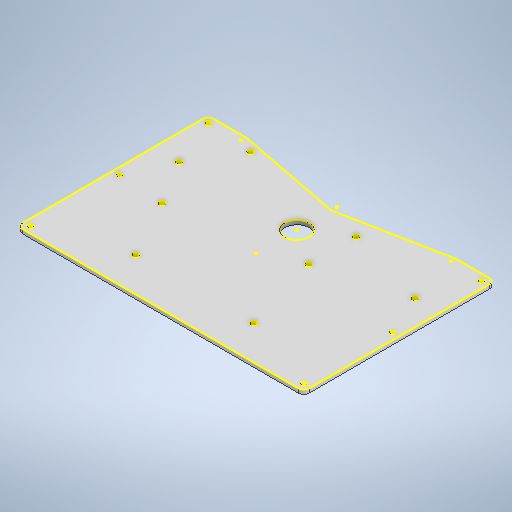
# Autodesk Inventor part: ローラー_板
Saved by Autodesk Inventor 2025.1 (Build 291241000, 241)
## iProperties
Created: 2024-10-14
Part Number: ローラー_板
Material: 一般
Document SubType Name: Modeling
Designer: taiju
Density: 1 g/cm^3
Appearance: 既定
Author: taiju
Autodesk Inventor part; units mm, degrees
ref_plane "YZ Plane" through (0, 0, 0) normal (1, 0, 0) x (0, 1, 0)
ref_plane "XZ Plane" through (0, 0, 0) normal (0, 1, 0) x (-1, 0, 0)
ref_plane "XY Plane" through (0, 0, 0) normal (0, 0, 1) x (1, 0, 0)
sketch "スケッチ1" plane through (0, 0, 0) normal (0, 1, 0) x (-1, 0, 0)
  line L0 (105, 70) -> (-105, 70)
  line L1 (-105, 70) -> (-105, -70)
  line L2 (-105, -70) -> (105, -70)
  line L3 (105, -70) -> (105, 70)
  line L4 (105, 70) -> (-105, -70) construction
  line L5 (-105, 70) -> (105, -70) construction
  circle A0 centre (0, -30) radius 77
  circle A1 centre (0, -30) radius 9
  line L6 (-105, -30) -> (105, -30)
  circle A2 centre (48, -30) radius 12.5
  circle A3 centre (-39, -30) radius 6
  circle A4 centre (48, -30) radius 17.5
  circle A5 centre (-39, -30) radius 9
  circle A6 centre (0, -30) radius 86.5
  line L7 (66.5, -30) -> (66.5, -62.5)
  line L8 (66.5, -30) -> (66.5, 2.5)
  line L9 (-26, -30) -> (-26, -47.5)
  line L10 (-26, -30) -> (-26, -12.5)
  circle A7 centre (65.5, -30) radius 2
  circle A8 centre (48, -12.5) radius 2
  circle A9 centre (30.5, -30) radius 2
  circle A10 centre (48, -47.5) radius 2
  circle A11 centre (-39, -39) radius 1.6
  circle A12 centre (-39, -21) radius 1.6
  circle A13 centre (-26, -47.5) radius 2
  circle A14 centre (-26, -12.5) radius 2
  circle A15 centre (66.5, -62.5) radius 2
  circle A16 centre (66.5, 2.5) radius 2
  circle A17 centre (86.5, -30) radius 2
  circle A18 centre (43.25, 44.9112) radius 2
  circle A19 centre (-43.25, 44.9112) radius 2
  circle A20 centre (-86.5, -30) radius 2
  line L11 (76.6958, -70) -> (0, -55)
  line L12 (0, -55) -> (-76.6958, -70)
  line L13 (100, -70) -> (100, 70)
  line L14 (-100, -70) -> (-100, 70)
  point P0 (0, 0)
  point P1 (-43.25, -104.9112)
  point P2 (43.25, -104.9112)
  point P3 (100, -65)
  point P4 (100, 0)
  point P5 (100, 65)
  point P6 (-100, -65)
  point P7 (-100, 0)
  point P8 (-100, 65)
  dimension "d9" = 35
  dimension "d0" = 210
  dimension "d1" = 140
  dimension "d2" = 100
  dimension "d3" = 154
  dimension "d4" = 18
  dimension "d5" = 48
  dimension "d6" = 39
  dimension "d7" = 25
  dimension "d8" = 12
  dimension "d10" = 18
  dimension "d11" = 173
  dimension "d14" = 360
  dimension "d16" = 18.5
  dimension "d17" = 32.5
  dimension "d18" = 32.5
  dimension "d20" = 13
  dimension "d21" = 17.5
  dimension "d22" = 17.5
  dimension "d25" = 360
  dimension "d27" = 4
  dimension "d28" = 4
  dimension "d29" = 4
  dimension "d30" = 4
  dimension "d31" = 3.2
  dimension "d32" = 3.2
  dimension "d33" = 4
  dimension "d34" = 4
  dimension "d35" = 4
  dimension "d36" = 4
  dimension "d37" = 4
  dimension "d38" = 4
  dimension "d39" = 4
  dimension "d40" = 4
  dimension "d41" = 15
  dimension "d45" = 5
  dimension "d46" = 5
  dimension "d47" = 5
  dimension "d48" = 5
  dimension "d49" = 5
  dimension "d50" = 5
  dimension "d51" = 5
  dimension "d52" = 5
  constraints: 30 end point, 26 coincident, 20 centre point, 17 point on line, 5 midpoint, 5 point on circle, 4 vertical, 2 parallel, 2 perpendicular, 1 horizontal, 1 horizontal alignment, 14 other
  measures "d0" distance of L2.end L1.end
  measures "d1" distance of L0.end L1.end
  measures "d2" distance from line of point (0, -30) L0
  measures "d3" diameter of A0
  measures "d4" diameter of A1
  measures "d5" distance of point (48, -30) point (0, -30)
  measures "d6" distance of point (-39, -30) point (0, -30)
  measures "d7" diameter of A2
  measures "d8" diameter of A3
  measures "d10" diameter of A5
  measures "d11" diameter of A6
  measures "d16" distance of L7.start point (48, -30)
  measures "d17" distance of L7.start L7.end
  measures "d18" distance of L7.start L8.end
  measures "d20" distance of L9.start A5.centre
  measures "d21" distance of L9.start L9.end
  measures "d22" distance of L9.start L10.end
  measures "d27" diameter of A7
  measures "d28" diameter of A8
  measures "d29" diameter of A9
  measures "d30" diameter of A10
  measures "d31" diameter of A11
  measures "d32" diameter of A12
  measures "d33" diameter of A13
  measures "d34" diameter of A14
  measures "d35" diameter of A15
  measures "d36" diameter of A16
  measures "d37" diameter of A17
  measures "d38" diameter of A18
  measures "d39" diameter of A19
  measures "d40" diameter of A20
  measures "d41" distance from line of L11.end L2
  measures "d45" distance from line of L13.start L3
  measures "d46" distance from line of L13.end L3
  measures "d47" distance from line of L14.start L1
  measures "d48" distance from line of L14.end L1
  measures "d49" distance from line of point (100, -65) L2
  measures "d50" distance from line of point (100, 65) L0
  measures "d51" distance from line of point (-100, -65) L2
  measures "d52" distance from line of point (-100, 65) L0
extrude "押し出し1" add sketch "スケッチ1" along normal blind 3 contours L3 L6 L13 L0 | L13 L6 A17 A6 A18 A19 A20 L14 L0 | L3 L2 L13 L6 | L14 L6 L1 L0 | L13 L2 A6 A17 L6 | L14 L2 L1 L6 | L6 A20 A6 L2 L14 | A17 L6 A0 A20 A6 A19 A18 | A6 L11 A0 L6 A17 | A20 L6 A0 L12 A6 | L11 L12 A0 L6 A5 A11 A1 A9 A4 A10 A7 | L6 A7 A4 A8 A9 A1 A5 A12 A0 | A7 L7 L6 | L6 L8 A7 | A5 A12 L6 A3 | L6 A3 A5 A11 | L7 A7 A4 L6 | L6 A4 A7 L8 | A3 L6 | L6 A3 | A12 A5 | A5 A12 | A11 A5 | A5 A11 | A4 A7 L6 | L6 A7 A4 | A7 L6 A2 A9 A4 A8 | A4 A10 A9 L6 A2 A7 | A8 A4 | A4 A8 | A10 A4 | A4 A10 | A2 L6 | L6 A2 | A9 L6 A4 | A4 L6 A9 | A9 L6 A4 | A4 L6 A9
fillet "フィレット1" radius 4 7 edges at (-105, 1.5, 70) (-105, 1.5, -70) (-76.6958, 1.5, -70) (0, 1.5, -55) (76.6958, 1.5, -70) (105, 1.5, -70) (105, 1.5, 70)
hole "穴1" at (-100, 0, 65) at (-100, 0, 0) at (-100, 0, -65) at (100, 0, -65) at (100, 0, 0) at (100, 0, 65) direction (0, 1, 0) diameter 3.2 end through all
sketch "スケッチ3" plane through (0, 3, 0) normal (0, 1, 0) x (1, 0, 0)
  circle A0 centre (100, -65) radius 1.6 projected
  circle A1 centre (100, 0) radius 1.6 projected
  circle A2 centre (100, 65) radius 1.6 projected
  circle A3 centre (-100, 65) radius 1.6 projected
  circle A4 centre (-100, 0) radius 1.6 projected
  circle A5 centre (-100, -65) radius 1.6 projected
  arc A6 (101, -70) -> (105, -66) centre (101, -66) ccw projected
  line L0 (105, -66) -> (105, 66) projected
  arc A7 (105, 66) -> (101, 70) centre (101, 66) ccw projected
  line L1 (101, 70) -> (77.0833, 70) projected
  arc A8 (77.0833, 70) -> (76.3155, 69.9256) centre (77.0833, 66) ccw projected
  line L2 (76.3155, 69.9256) -> (0.7678, 55.1502) projected
  arc A9 (-0.7678, 55.1502) -> (0.7678, 55.1502) centre (0, 59.0758) ccw projected
  line L3 (-0.7678, 55.1502) -> (-76.3155, 69.9256) projected
  arc A10 (-76.3155, 69.9256) -> (-77.0833, 70) centre (-77.0833, 66) ccw projected
  line L4 (-77.0833, 70) -> (-101, 70) projected
  arc A11 (-101, 70) -> (-105, 66) centre (-101, 66) ccw projected
  line L5 (-105, 66) -> (-105, -66) projected
  arc A12 (-105, -66) -> (-101, -70) centre (-101, -66) ccw projected
  line L6 (-101, -70) -> (101, -70) projected
  circle A13 centre (43.25, -44.9112) radius 2 projected
  circle A14 centre (-43.25, -44.9112) radius 2 projected
  circle A15 centre (-86.5, 30) radius 2 projected
  circle A16 centre (-66.5, 62.5) radius 2 projected
  circle A17 centre (-66.5, -2.5) radius 2 projected
  circle A18 centre (0, 30) radius 9 projected
  circle A19 centre (26, 47.5) radius 2 projected
  circle A20 centre (26, 12.5) radius 2 projected
  circle A21 centre (86.5, 30) radius 2 projected
  point P0 (0, 0)
